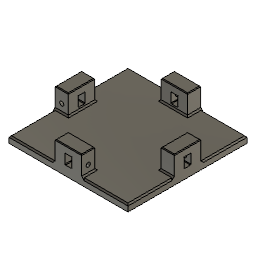
fixation plate final assempbly (Autodesk Fusion 360 archive; units mm, degrees)
design "fixation plate"
part number: 2026-04-10-15-32-10-138
Autodesk Fusion 360 part; units mm, degrees
sketch "Sketch1" plane through (0, 0, 0) normal (0, 0, 1) x (1, 0, 0)
  line L0 (-160.2344, 10.4731) -> (19.7656, 10.4731)
  line L1 (19.7656, 10.4731) -> (19.7656, -169.5269)
  line L2 (19.7656, -169.5269) -> (-160.2344, -169.5269)
  line L3 (-160.2344, -169.5269) -> (-160.2344, 10.4731)
  dimension "d1" = 180
  dimension "d2" = 180
  constraint horizontal L0
  constraint vertical L1
  constraint horizontal L2
  constraint vertical L3
  measures "d1" distance of L1 L3
  measures "d2" distance of L0 L2
extrude "Extrude1" add sketch "Sketch1" along normal blind 10
sketch "Sketch2" plane through (0, 0, 10) normal (0, 0, 1) x (-1, 0, 0)
  line L0 (160.2344, 169.5269) -> (-19.7656, 169.5269)
  line L1 (-19.7656, 169.5269) -> (-19.7656, -10.4731)
  line L2 (-19.7656, -10.4731) -> (160.2344, -10.4731)
  line L3 (160.2344, -10.4731) -> (160.2344, 169.5269)
  line L4 (160.2344, 59.5269) -> (140.2344, 59.5269)
  line L5 (140.2344, 59.5269) -> (140.2344, 99.5269)
  line L6 (140.2344, 99.5269) -> (160.2344, 99.5269)
  line L7 (160.2344, 99.5269) -> (160.2344, 59.5269)
  line L8 (0.2344, 59.5269) -> (-19.7656, 59.5269)
  line L9 (-19.7656, 59.5269) -> (-19.7656, 99.5269)
  line L10 (-19.7656, 99.5269) -> (0.2344, 99.5269)
  line L11 (0.2344, 99.5269) -> (0.2344, 59.5269)
  line L12 (90.2344, -10.4731) -> (50.2344, -10.4731)
  line L13 (50.2344, -10.4731) -> (50.2344, 9.5269)
  line L14 (50.2344, 9.5269) -> (90.2344, 9.5269)
  line L15 (90.2344, 9.5269) -> (90.2344, -10.4731)
  line L16 (90.2344, 149.5269) -> (50.2344, 149.5269)
  line L17 (50.2344, 149.5269) -> (50.2344, 169.5269)
  line L18 (50.2344, 169.5269) -> (90.2344, 169.5269)
  line L19 (90.2344, 169.5269) -> (90.2344, 149.5269)
  dimension "d5" = 20
  dimension "d6" = 20
  dimension "d7" = 20
  dimension "d8" = 20
  dimension "d9" = 40
  dimension "d10" = 40
  dimension "d11" = 40
  dimension "d12" = 40
  dimension "d13" = 70
  dimension "d14" = 70
  dimension "d15" = 70
  dimension "d16" = 70
  constraint horizontal L4
  constraint vertical L5
  constraint horizontal L6
  constraint vertical L7
  constraint horizontal L8
  constraint vertical L9
  constraint horizontal L10
  constraint vertical L11
  constraint horizontal L12
  constraint vertical L13
  constraint horizontal L14
  constraint vertical L15
  constraint horizontal L16
  constraint vertical L17
  constraint horizontal L18
  constraint vertical L19
  constraint collinear L3 L7
  constraint collinear L2 L12
  constraint collinear L1 L9
  constraint collinear L0 L18
  measures "d5" distance of L16 L18
  measures "d6" distance of L9 L11
  measures "d7" distance of L12 L14
  measures "d8" distance of L5 L7
  measures "d9" distance of L4 L6
  measures "d10" distance of L8 L10
  measures "d11" distance of L13 L15
  measures "d12" distance of L17 L19
  measures "d13" distance of L2 L4
  measures "d14" distance of L3 L19
  measures "d15" distance of L2 L8
  measures "d16" distance of L3 L15
extrude "Extrude2" add sketch "Sketch2" along normal blind 30 contours L0 L16 L17 L18 L19 | L3 L4 L5 L6 L7 | L1 L8 L9 L10 L11 | L2 L12 L13 L14 L15
sketch "Sketch3" plane through (19.7656, 0, 0) normal (1, 0, 0) x (0, 1, 0)
  line L0 (-169.5269, 0) -> (10.4731, 0)
  line L1 (10.4731, 0) -> (10.4731, 10)
  line L2 (10.4731, 10) -> (-59.5269, 10)
  line L3 (-59.5269, 10) -> (-59.5269, 40)
  line L4 (-59.5269, 40) -> (-99.5269, 40)
  line L5 (-99.5269, 40) -> (-99.5269, 10)
  line L6 (-99.5269, 10) -> (-169.5269, 10)
  line L7 (-169.5269, 10) -> (-169.5269, 0)
  circle A0 centre (-79.5269, 22) radius 6 construction
  line L8 (-74.5269, 29.5) -> (-84.5269, 29.5) construction
  line L9 (-84.5269, 29.5) -> (-84.5269, 15.25) construction
  line L10 (-83.7769, 14.5) -> (-75.2769, 14.5) construction
  line L11 (-74.5269, 15.25) -> (-74.5269, 29.5) construction
  line L12 (-74.5269, 29.5) -> (-84.5269, 14.5) construction
  line L13 (-84.5269, 29.5) -> (-74.5269, 14.5) construction
  line L14 (-83.7769, 14.5) -> (-84.5269, 15.25)
  line L15 (-75.2769, 14.5) -> (-74.5269, 15.25)
  line L16 (-83.839, 14.35) -> (-75.2147, 14.35)
  line L17 (-75.2147, 14.35) -> (-74.3769, 15.1879)
  line L18 (-74.3769, 15.1879) -> (-74.3769, 29.65)
  line L19 (-74.3769, 29.65) -> (-84.6769, 29.65)
  line L20 (-84.6769, 29.65) -> (-84.6769, 15.1879)
  line L21 (-83.839, 14.35) -> (-84.6769, 15.1879)
  point P0 (-79.5269, 22)
  dimension "d19" = 12
  dimension "d20" = 18
  dimension "d21" = 20
  dimension "d36" = 10
  dimension "d37" = 15
  dimension "d38" = 0.15
  dimension "d39" = 0.75
  dimension "d40" = 0.75
  dimension "d41" = 0.75
  dimension "d42" = 0.75
  constraint horizontal L8
  constraint perpendicular L8 L9
  constraint parallel L8 L10
  constraint parallel L9 L11
  constraint coincident L12 P0
  constraint coincident L13 P0
  constraint coincident P0 A0.centre
  constraint coincident L12.end L10
  constraint coincident L12.end L9
  constraint coincident L13.end L10
  constraint coincident L13.end L11
  measures "d19" diameter of A0
  measures "d20" distance of L4 P0
  measures "d21" distance of L5 P0
  measures "d36" distance of L12.end L13.end
  measures "d37" distance of L8.end L12.end
  measures "d39" distance of L12.end L10.start
  measures "d40" distance of L12.end L9.end
  measures "d41" distance of L13.end L10.end
  measures "d42" distance of L13.end L11.start
extrude "Extrude3" cut sketch "Sketch3" against normal blind 30 contours L16 L17 L18 L19 L20 L21
ref_plane "WorkPlane1" through (-70.2344, -79.5269, 20) normal (0, -1, 0) x (1, 0, 0)
ref_plane "WorkPlane2" through (-70.2344, -79.5269, 20) normal (1, 0, 0) x (0, 1, 0)
pattern_circular "C-Pattern1" count 4 over 360 about axis through (-70.2344, -79.5269, -13.6) along (0, 0, 1) of "Extrude3"
sketch "Sketch4" plane through (0, -59.5269, 0) normal (0, 1, 0) x (-1, 0, 0)
  line L0 (-19.7656, 10) -> (0.2344, 10)
  line L1 (0.2344, 10) -> (0.2344, 40)
  line L2 (0.2344, 40) -> (-19.7656, 40)
  line L3 (-19.7656, 40) -> (-19.7656, 10)
  circle A0 centre (-9.7656, 22) radius 3.1
  dimension "d26" = 6.2
  dimension "d27" = 18
  dimension "d28" = 10
  measures "d26" diameter of A0
  measures "d27" distance of L2 A0.centre
  measures "d28" distance of L3 A0.centre
extrude "Extrude4" cut sketch "Sketch4" against normal blind 20 contours A0
pattern_circular "C-Pattern2" count 4 over 360 about axis through (-70.2344, -79.5269, -13.6) along (0, 0, 1) of "Extrude4"
chamfer "Chamfer1" distance 1 angle 45 16 edges at (-0.2344, -79.5269, 40) (9.7656, -99.5269, 40) (19.7656, -79.5269, 40) (9.7656, -59.5269, 40) (-70.2344, 10.4731, 40) (-70.2344, -9.5269, 40) (-50.2344, 0.4731, 40) (-90.2344, 0.4731, 40) (-150.2344, -59.5269, 40) (-140.2344, -79.5269, 40) (-160.2344, -79.5269, 40) (-150.2344, -99.5269, 40) (-90.2344, -159.5269, 40) (-70.2344, -149.5269, 40) (-70.2344, -169.5269, 40) (-50.2344, -159.5269, 40)
chamfer "Chamfer2" distance 2 angle 45 12 edges at (-140.2344, -79.5269, 10) (-150.2344, -99.5269, 10) (-150.2344, -59.5269, 10) (-70.2344, -149.5269, 10) (-90.2344, -159.5269, 10) (-90.2344, 0.4731, 10) (-70.2344, -9.5269, 10) (-0.2344, -79.5269, 10) (9.7656, -99.5269, 10) (-50.2344, -159.5269, 10) (9.7656, -59.5269, 10) (-50.2344, 0.4731, 10)
chamfer "Chamfer3" distance 2 angle 45 8 edges at (-126.2344, 10.4731, 10) (-160.2344, -23.5269, 10) (19.7656, -23.5269, 10) (19.7656, -135.5269, 10) (-14.2344, -169.5269, 10) (-14.2344, 10.4731, 10) (-126.2344, -169.5269, 10) (-160.2344, -135.5269, 10)
equation "d40 = d39"
equation "d42 = d41"
